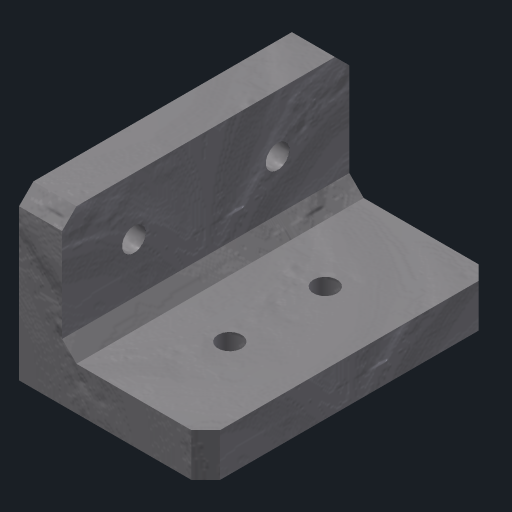
# Autodesk Inventor part: SOPORTE_TOBOGAN_V2
Saved by Autodesk Inventor 2024.3 (Build 283343000, 343)
## iProperties
Created: 2024-09-04
Part Number: SOPORTE_TOBOGAN_V2
Material: Steel, Mild, Welded
Document SubType Name: Modeling
Designer: Niler
Density: 7.85 g/cm^3
Appearance: Weld - Steel Mild
Author: Niler
Autodesk Inventor part; units mm, degrees
ref_plane "YZ Plane" through (0, 0, 0) normal (1, 0, 0) x (0, 1, 0)
ref_plane "XZ Plane" through (0, 0, 0) normal (0, 1, 0) x (-1, 0, 0)
ref_plane "XY Plane" through (0, 0, 0) normal (0, 0, 1) x (1, 0, 0)
sketch "Sketch1" plane through (0, 0, 0) normal (1, 0, 0) x (0, 1, 0)
  circle A0 centre (15, 10) radius 1.65
  line L0 (0, 0) -> (9.4364, 0)
  circle A1 centre (15, -10) radius 1.65
  line L1 (0, 20) -> (23, 20)
  line L2 (23, 20) -> (23, -20)
  line L3 (23, -20) -> (0, -20)
  line L4 (0, -20) -> (0, 20)
  dimension "d0" = 15
  dimension "d1" = 20
  dimension "d2" = 3.3
  dimension "d3" = 23
  dimension "d4" = 40
  constraints: 10 end point, 2 centre point, 2 horizontal, 2 parallel, 1 midpoint, 1 perpendicular, 1 symmetric about line, 1 other
  measures "d0" horizontal distance of L0.start A0.centre
  measures "d1" distance of A1.centre A0.centre
  measures "d2" diameter of A0
  measures "d3" distance of L2.end L3.end
  measures "d4" distance of L3.end L1.start
extrude "Extrusion1" add sketch "Sketch1" along normal blind 6
sketch "Sketch2" plane through (6, 0, 0) normal (1, 0, 0) x (0, 0, -1)
  line L0 (20, 23) -> (-20, 23) projected
  line L1 (-20, 23) -> (-20, 0) projected
  line L2 (-20, 0) -> (20, 0) projected
  line L3 (20, 0) -> (20, 23) projected
  circle A0 centre (-10, 15) radius 1.65 projected
  circle A1 centre (10, 15) radius 1.65 projected
  line L4 (-20, 0) -> (20, 0)
  line L5 (20, 0) -> (20, 6)
  line L6 (20, 6) -> (-20, 6)
  line L7 (-20, 6) -> (-20, 0)
  point P0 (0, 0)
  dimension "d7" = 6
  constraints: 8 end point, 2 parallel, 1 horizontal, 1 perpendicular, 1 point on line
  measures "d7" distance between parallel lines of L2 L6
extrude "Extrusion2" add sketch "Sketch2" along normal blind 20 contours L3 L2 L1 L6
sketch "Sketch3" plane through (6, 6, 20) normal (0, 1, 0) x (1, 0, 0)
  line L0 (0, 0) -> (0, 40) projected
  line L1 (0, 0) -> (20, 0) projected
  line L2 (20, 40) -> (20, 0) projected
  line L3 (0, 40) -> (20, 40) projected
  circle A0 centre (10, 13.35) radius 1.65
  circle A1 centre (10, 26.65) radius 1.65
  line L4 (10, 13.35) -> (10, 26.65) construction
  point P0 (-6, 20)
  point P1 (10, 40)
  point P2 (10, 20)
  point P3 (0, 20)
  dimension "d10" = 3.3
  dimension "d11" = 10
  constraints: 3 midpoint, 2 centre point, 2 end point, 2 vertical alignment, 1 equal radius, 1 horizontal alignment, 1 vertical
  measures "d10" diameter of A0
extrude "Extrusion3" cut sketch "Sketch3" against normal through all contours A0 | A1
chamfer "Chamfer1" distance 2 angle 45 5 edges at (3, 23, 20) (3, 23, -20) (26, 3, 20) (26, 3, -20) (6, 6, 0)
body "Solid1"
